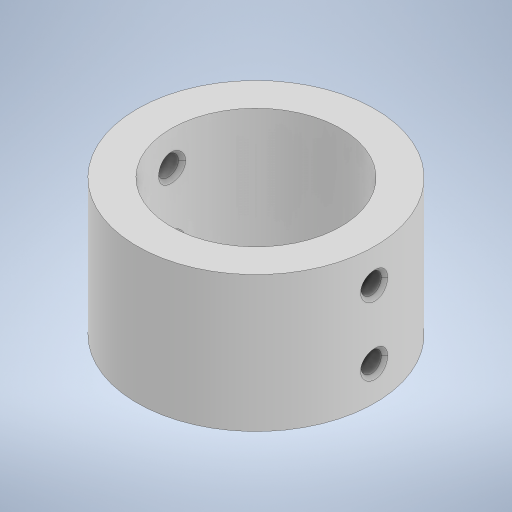
# Autodesk Inventor part: Муфта ограничителя шкива
Saved by Autodesk Inventor 2023 (Build 270158000, 158)
## iProperties
Created: 2022-05-17
Part Number: Муфта ограничителя шкива
Material: Типовые
Document SubType Name: Modeling
Designer: avkap
Density: 1 g/cm^3
Appearance: По умолчанию
Author: avkap
Autodesk Inventor part; units mm, degrees
ref_plane "YZ Plane" through (0, 0, 0) normal (1, 0, 0) x (0, 1, 0)
ref_plane "XZ Plane" through (0, 0, 0) normal (0, 1, 0) x (-1, 0, 0)
ref_plane "XY Plane" through (0, 0, 0) normal (0, 0, 1) x (1, 0, 0)
sketch "Эскиз1" plane through (0, 0, 0) normal (0, 1, 0) x (-1, 0, 0)
  circle A0 centre (0, 0) radius 12.5
  circle A1 centre (0, 0) radius 17.5
  dimension "d0" = 25
  dimension "d1" = 35
  constraints: 2 centre point, 2 coincident
  measures "d0" diameter of A0
  measures "d1" diameter of A1
extrude "Выдавливание1" add sketch "Эскиз1" along normal blind 20
sketch "Эскиз2" plane through (0, 0, 0) normal (1, 0, 0) x (0, 1, 0)
  line L0 (20, -17.5) -> (20, 17.5) projected
  line L1 (20, 0) -> (15, 0)
  circle A0 centre (15, 0) radius 1.5
  line L2 (15, 0) -> (5, 0)
  circle A1 centre (5, 0) radius 1.5
  point P0 (0, 0)
  dimension "d4" = 5
  dimension "d5" = 3
  dimension "d11" = 10
  dimension "d12" = 3
  constraints: 4 end point, 2 centre point, 2 coincident, 2 horizontal, 1 midpoint
  measures "d4" distance of L1.start L1.end
  measures "d5" diameter of A0
  measures "d11" distance of L2.start L2.end
  measures "d12" diameter of A1
extrude "Выдавливание2" cut sketch "Эскиз2" along normal mid plane 56.5
chamfer "Фаска1" distance 0.5 angle 45 12 edges at (-12.4097, 15.0001, 1.5) (-12.4097, 15.0013, -1.5) (12.5, 13.5001, -0.0192) (-17.4356, 15.0001, 1.5) (-17.4356, 15, -1.5) (17.5, 13.5001, -0.0201) (-17.4356, 5.0001, 1.5) (-17.4356, 5, -1.5) (17.5, 3.5001, -0.0201) (-12.4097, 5.0001, 1.5) (-12.4097, 5.0013, -1.5) (12.5, 3.5001, -0.0192)
